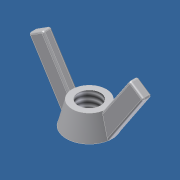
# Autodesk Inventor part: HW-00011
Saved by Autodesk Inventor 2011 (Build 150239000, 239)
## iProperties
Created: 2008-05-30
Part Number: HW-00011
Document SubType Name: Modeling
Designer: mcyr
Density: 1 g/cm^3
Description: 1/4-20 Wing Nut
Mass: 0.395364 g
Surface Area: 6.11507 cm^2
Volume: 0.395364 cm^3
Author: mcyr
Autodesk Inventor part; units mm, degrees
ref_plane "YZ Plane" through (0, 0, 0) normal (1, 0, 0) x (0, 1, 0)
ref_plane "XZ Plane" through (0, 0, 0) normal (0, 1, 0) x (-1, 0, 0)
ref_plane "XY Plane" through (0, 0, 0) normal (0, 0, 1) x (1, 0, 0)
sketch "Sketch1" plane through (0, 0, 0) normal (0, 0, 1) x (1, 0, 0)
  line L0 (2.4697, 4.4922) -> (-2.6103, 4.4922)
  line L1 (-2.6103, 4.4922) -> (-1.3403, 9.5722)
  line L2 (-1.3403, 9.5722) -> (2.4697, 9.5722)
  line L3 (2.4697, 9.5722) -> (2.4697, 4.4922)
  line L4 (7.5497, 4.4922) -> (6.2797, 9.5722)
  line L5 (-2.6103, 4.4922) -> (-10.1562, 16.4603)
  line L6 (-10.1562, 16.4603) -> (-6.9812, 18.4622)
  line L7 (-6.9812, 18.4622) -> (-1.3403, 9.5722)
  line L8 (7.5497, 4.4922) -> (15.4912, 16.3327)
  line L9 (15.4912, 16.3327) -> (12.3162, 18.4622)
  line L10 (12.3162, 18.4622) -> (6.2797, 9.5722)
  dimension "d0" = 3.175
  dimension "d1" = 3.175
  dimension "d3" = 3.81
  dimension "d4" = 5.08
  dimension "d5" = 5.08
  dimension "d6" = 5.08
  dimension "d8" = 13.97
  dimension "d9" = 13.97
  constraints: 22 end point, 3 perpendicular, 1 horizontal, 1 parallel
  measures "d0" horizontal distance of L5.end L6.end
  measures "d1" horizontal distance of L8.end L9.end
  measures "d3" distance of L1.end L2.end
  measures "d4" distance of L0.start L0.end
  measures "d5" vertical distance of L0.end L1.end
  measures "d6" vertical distance of L4.start L4.end
  measures "d8" vertical distance of L4.start L9.end
  measures "d9" vertical distance of L0.end L6.end
revolve "Revolution1" add sketch "Sketch1" angle 360 about axis through (2.4697, 9.5722, 0) along (0, -1, 0) contours L0 L1 L2 L3
extrude "Extrusion1" add sketch "Sketch1" along normal mid plane 1.905 contours L5 L6 L7 L1
extrude "Extrusion2" add sketch "Sketch1" along normal mid plane 1.905 contours L4 L10 L9 L8
fillet "Fillet1" radius 0.381 16 edges at (-6.3833, 10.4762, 0.9525) (-4.1608, 14.0172, 0.9525) (-4.1608, 14.0172, -0.9525) (9.2979, 14.0172, 0.9525) (12.3162, 18.4622, 0) (9.2979, 14.0172, -0.9525) (13.9037, 17.3974, -0.9525) (13.9037, 17.3974, 0.9525) (15.4912, 16.3327, 0) (11.5204, 10.4124, -0.9525) (11.5204, 10.4124, 0.9525) (-8.5687, 17.4612, 0.9525) (-10.1562, 16.4603, 0) (-8.5687, 17.4612, -0.9525) (-6.9812, 18.4622, 0) (-6.3833, 10.4762, -0.9525)
hole "Hole1" at (2.4697, 9.5722, 0) direction (0, -1, 0) diameter 4.9784 depth 19.05 tip angle 118 thread size "1/4-20 UNC" class "2B" standard "ANSI Unified Screw Threads"
body "Solid1"
